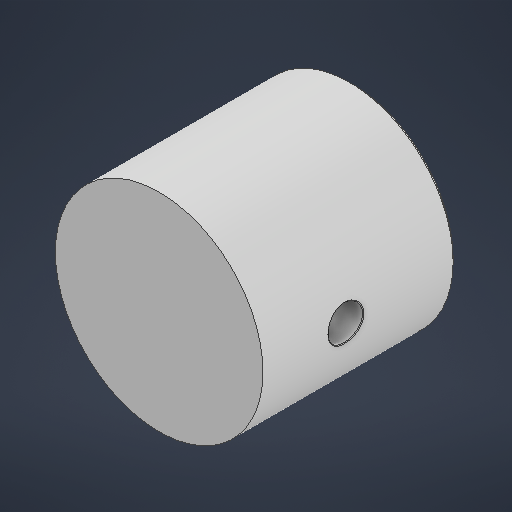
# Autodesk Inventor part: Piston
Saved by Autodesk Inventor 2025.4 (Build 294407000, 407)
## iProperties
Created: 2026-05-29
Part Number: Piston
Material: Generic
Document SubType Name: Modeling
Designer: VuQuan
Density: 1 g/cm^3
Appearance: Default
Author: VuQuan
Autodesk Inventor part; units mm, degrees
ref_plane "YZ Plane" through (0, 0, 0) normal (1, 0, 0) x (0, 1, 0)
ref_plane "XZ Plane" through (0, 0, 0) normal (0, 1, 0) x (-1, 0, 0)
ref_plane "XY Plane" through (0, 0, 0) normal (0, 0, 1) x (1, 0, 0)
sketch "Sketch1" plane through (0, 0, 0) normal (0, 0, 1) x (1, 0, 0)
  circle A0 centre (0, 0) radius 10
  circle A1 centre (0, 0) radius 11
  circle A2 centre (0, 0) radius 15
  dimension "d0" = 20
  dimension "d1" = 22
  dimension "d2" = 30
  constraints: 3 centre point, 3 coincident
  measures "d0" diameter of A0
  measures "d1" diameter of A1
  measures "d2" diameter of A2
extrude "Extrusion1" add sketch "Sketch1" along normal blind 28 contours A0 | A1 | A2
extrude "Extrusion2" cut sketch "Sketch1" along normal blind 12 contours A1
extrude "Extrusion3" cut sketch "Sketch1" along normal blind 27 contours A0
sketch "Sketch2" plane through (0, 0, 0) normal (1, 0, 0) x (0, 1, 0)
  line L0 (15, 28) -> (-15, 28) projected
  line L1 (15, 0) -> (-15, 0) projected
  circle A0 centre (0, 16) radius 2.5
  point P0 (0, 0)
  point P1 (0, 0)
  dimension "d9" = 5
  dimension "d10" = 16
  constraints: 1 centre point, 1 coincident, 1 midpoint, 1 vertical alignment
  measures "d9" diameter of A0
  measures "d10" distance from line of L1 A0.centre
extrude "Extrusion4" cut sketch "Sketch2" along normal through all both and the other way through all
chamfer "Chamfer1" distance 0.5 angle 45 2 edges at (-11, 0, 0) (-15, 0, 0)
chamfer "Chamfer2" distance 0.1 angle 45 4 edges at (14.7902, -2.5, 16.0004) (14.8791, 1.901, 14.3764) (14.8788, 1.9027, 17.6217) (-14.7902, -2.4999, 15.9815)
body "Solid1"
